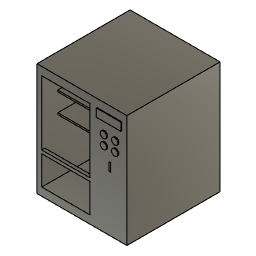
vendmachineprototype (Autodesk Fusion 360 design; units mm, degrees)
Autodesk Fusion 360 part; units mm, degrees
sketch "Sketch1" plane through (0, 0, 0) normal (0, 0, 1) x (1, 0, 0)
  line L0 (140, -145) -> (-140, -145)
  line L1 (-140, -145) -> (-140, 145)
  line L2 (-140, 145) -> (140, 145)
  line L3 (140, 145) -> (140, -145)
  line L4 (140, -145) -> (-140, 145) construction
  line L5 (-140, -145) -> (140, 145) construction
  dimension "d1" = 280
  dimension "d2" = 290
  constraint horizontal L0
  constraint perpendicular L0 L1
  constraint parallel L0 L2
  constraint parallel L1 L3
  constraint coincident L4 origin
  constraint coincident L5 origin
  measures "d1" distance of L1.end L2.end
  measures "d2" distance of L0.end L1.end
extrude "Extrude1" add sketch "Sketch1" along normal blind 350
sketch "Sketch2" plane through (0, -145, 0) normal (0, -1, 0) x (1, 0, 0)
  line L0 (-140, 0) -> (140, 0)
  line L1 (140, 0) -> (140, 350)
  line L2 (140, 350) -> (-140, 350)
  line L3 (-140, 350) -> (-140, 0)
  line L4 (25, 125) -> (-125, 125)
  line L5 (-125, 125) -> (-125, 325)
  line L6 (-125, 325) -> (25, 325)
  line L7 (25, 325) -> (25, 125)
  line L8 (25, 125) -> (-125, 325) construction
  line L9 (-125, 125) -> (25, 325) construction
  point P0 (-50, 225)
  constraint horizontal L4
  constraint perpendicular L4 L5
  constraint parallel L4 L6
  constraint parallel L5 L7
  constraint coincident L8 P0
  constraint coincident L9 P0
extrude "Extrude2" cut sketch "Sketch2" against normal blind 200 contours L4 L5 L6 L7
sketch "Sketch3" plane through (0, -145, 0) normal (0, -1, 0) x (1, 0, 0)
  line L0 (-125, 125) -> (-125, 325)
  line L1 (-125, 325) -> (25, 325)
  line L2 (25, 325) -> (25, 125)
  line L3 (25, 125) -> (-125, 125)
  line L4 (-140, 0) -> (140, 0)
  line L5 (140, 0) -> (140, 350)
  line L6 (140, 350) -> (-140, 350)
  line L7 (-140, 350) -> (-140, 0)
  line L8 (123.6698, 300.3073) -> (46.6698, 300.3073)
  line L9 (46.6698, 300.3073) -> (46.6698, 325.3073)
  line L10 (46.6698, 325.3073) -> (123.6698, 325.3073)
  line L11 (123.6698, 325.3073) -> (123.6698, 300.3073)
  line L12 (123.6698, 300.3073) -> (46.6698, 325.3073) construction
  line L13 (46.6698, 300.3073) -> (123.6698, 325.3073) construction
  circle A0 centre (70, 260) radius 9
  circle A1 centre (100, 260) radius 9
  circle A2 centre (70, 230) radius 9
  circle A3 centre (100, 230) radius 9
  line L14 (25, 22.9549) -> (-125, 22.9549)
  line L15 (-125, 22.9549) -> (-125, 112.9549)
  line L16 (-125, 112.9549) -> (25, 112.9549)
  line L17 (25, 112.9549) -> (25, 22.9549)
  line L18 (25, 22.9549) -> (-125, 112.9549) construction
  line L19 (-125, 22.9549) -> (25, 112.9549) construction
  line L20 (85, 185) -> (95, 185)
  line L21 (95, 185) -> (95, 160)
  line L22 (95, 160) -> (85, 160)
  line L23 (85, 160) -> (85, 185)
  point P0 (85.1698, 312.8073)
  point P1 (-50, 67.9549)
  dimension "d7" = 77
  dimension "d8" = 25
  dimension "d9" = 18
  dimension "d10" = 18
  dimension "d11" = 18
  dimension "d12" = 18
  dimension "d13" = 150
  dimension "d14" = 90
  constraint horizontal L8
  constraint perpendicular L8 L9
  constraint parallel L8 L10
  constraint parallel L9 L11
  constraint coincident L12 P0
  constraint coincident L13 P0
  constraint horizontal L14
  constraint perpendicular L14 L15
  constraint parallel L14 L16
  constraint parallel L15 L17
  constraint coincident L18 P1
  constraint coincident L19 P1
  constraint horizontal L20
  constraint vertical L21
  constraint horizontal L22
  constraint vertical L23
  measures "d7" distance of L9.end L10.end
  measures "d8" distance of L8.end L9.end
  measures "d9" diameter of A0
  measures "d10" diameter of A1
  measures "d11" diameter of A2
  measures "d12" diameter of A3
  measures "d13" distance of L15.end L16.end
  measures "d14" distance of L14.end L15.end
extrude "Extrude3" add sketch "Sketch3" along normal blind 2 contours L8 L9 L10 L11
sketch "Sketch4" plane through (0, 55, 0) normal (0, -1, 0) x (1, 0, 0)
  line L0 (25, 325) -> (-125, 325)
  line L1 (-125, 325) -> (-125, 125)
  line L2 (-125, 125) -> (25, 125)
  line L3 (25, 125) -> (25, 325)
  line L4 (-125, 200.3816) -> (25, 200.3816)
  line L5 (25, 200.3816) -> (25, 195.3816)
  line L6 (25, 195.3816) -> (-125, 195.3816)
  line L7 (-125, 195.3816) -> (-125, 200.3816)
  line L8 (-125, 261.7004) -> (25, 261.7004)
  line L9 (25, 261.7004) -> (25, 256.7004)
  line L10 (25, 256.7004) -> (-125, 256.7004)
  line L11 (-125, 256.7004) -> (-125, 261.7004)
  dimension "d17" = 5
  dimension "d18" = 150
  dimension "d19" = 5
  constraint horizontal L4
  constraint vertical L5
  constraint horizontal L6
  constraint vertical L7
  constraint coincident L1 L4.start
  constraint horizontal L8
  constraint vertical L9
  constraint horizontal L10
  constraint vertical L11
  constraint coincident L1 L8.start
  measures "d17" distance of L4.start L6.end
  measures "d18" distance of L8.start L8.end
  measures "d19" distance of L8.start L10.end
extrude "Extrude4" add sketch "Sketch4" along normal blind 150 contours L1 L3 L8 L9 L10 L11 | L1 L3 L4 L5 L6 L7
sketch "Sketch5" plane through (0, 0, 125) normal (0, 0, 1) x (-1, 0, 0)
  line L0 (125, 145) -> (-25, 145)
  line L1 (-25, 145) -> (-25, -55)
  line L2 (-25, -55) -> (125, -55)
  line L3 (125, -55) -> (125, 145)
  line L4 (-25, 135) -> (125, 135)
  line L5 (125, 135) -> (125, 5)
  line L6 (125, 5) -> (-25, 5)
  line L7 (-25, 5) -> (-25, 135)
  line L8 (-25, 135) -> (125, 5) construction
  line L9 (125, 135) -> (-25, 5) construction
  point P0 (50, 70)
  dimension "d22" = 130
  constraint horizontal L4
  constraint perpendicular L4 L5
  constraint parallel L4 L6
  constraint parallel L5 L7
  constraint coincident L8 P0
  constraint coincident L9 P0
  measures "d22" distance of L4.end L5.end
extrude "Extrude5" cut sketch "Sketch5" against normal blind 75 contours L1 L3 L4 L5 L6 L7
sketch "Sketch6" plane through (0, -145, 0) normal (0, -1, 0) x (1, 0, 0)
  line L0 (123.6698, 325.3073) -> (123.6698, 300.3073)
  line L1 (123.6698, 300.3073) -> (46.6698, 300.3073)
  line L2 (46.6698, 300.3073) -> (46.6698, 325.3073)
  line L3 (46.6698, 325.3073) -> (123.6698, 325.3073)
  line L4 (-125, 125) -> (-125, 325)
  line L5 (-125, 325) -> (25, 325)
  line L6 (25, 325) -> (25, 125)
  line L7 (25, 125) -> (-125, 125)
  line L8 (-140, 0) -> (140, 0)
  line L9 (140, 0) -> (140, 350)
  line L10 (140, 350) -> (-140, 350)
  line L11 (-140, 350) -> (-140, 0)
  line L12 (25, 25) -> (-125, 25)
  line L13 (-125, 25) -> (-125, 115)
  line L14 (-125, 115) -> (25, 115)
  line L15 (25, 115) -> (25, 25)
  line L16 (25, 25) -> (-125, 115) construction
  line L17 (-125, 25) -> (25, 115) construction
  point P0 (-50, 70)
  dimension "d25" = 150
  dimension "d26" = 90
  constraint horizontal L12
  constraint perpendicular L12 L13
  constraint parallel L12 L14
  constraint parallel L13 L15
  constraint coincident L16 P0
  constraint coincident L17 P0
  measures "d25" distance of L13.end L14.end
  measures "d26" distance of L12.end L13.end
extrude "Extrude6" cut sketch "Sketch6" against normal blind 150 contours L12 L13 L14 L15
sketch "Sketch7" plane through (0, -145, 0) normal (0, -1, 0) x (1, 0, 0)
  line L0 (-125, 25) -> (-125, 115)
  line L1 (-125, 115) -> (25, 115)
  line L2 (25, 115) -> (25, 25)
  line L3 (25, 25) -> (-125, 25)
  line L4 (123.6698, 325.3073) -> (123.6698, 300.3073)
  line L5 (123.6698, 300.3073) -> (46.6698, 300.3073)
  line L6 (46.6698, 300.3073) -> (46.6698, 325.3073)
  line L7 (46.6698, 325.3073) -> (123.6698, 325.3073)
  line L8 (-125, 125) -> (-125, 325)
  line L9 (-125, 325) -> (25, 325)
  line L10 (25, 325) -> (25, 125)
  line L11 (25, 125) -> (-125, 125)
  line L12 (-140, 0) -> (140, 0)
  line L13 (140, 0) -> (140, 350)
  line L14 (140, 350) -> (-140, 350)
  line L15 (-140, 350) -> (-140, 0)
  circle A0 centre (70, 265) radius 10
  circle A1 centre (105, 265) radius 10
  circle A2 centre (70, 235) radius 10
  circle A3 centre (105, 235) radius 10
  dimension "d29" = 20
  dimension "d30" = 20
  dimension "d31" = 20
  dimension "d32" = 20
  measures "d29" diameter of A0
  measures "d30" diameter of A1
  measures "d31" diameter of A2
  measures "d32" diameter of A3
extrude "Extrude7" add sketch "Sketch7" along normal blind 3 contours A0 | A1 | A2 | A3
sketch "Sketch8" plane through (0, -145, 0) normal (0, -1, 0) x (1, 0, 0)
  circle A0 centre (105, 235) radius 10
  circle A1 centre (70, 265) radius 10
  circle A2 centre (70, 235) radius 10
  circle A3 centre (105, 265) radius 10
  line L0 (-125, 25) -> (-125, 115)
  line L1 (-125, 115) -> (25, 115)
  line L2 (25, 115) -> (25, 25)
  line L3 (25, 25) -> (-125, 25)
  line L4 (123.6698, 325.3073) -> (123.6698, 300.3073)
  line L5 (123.6698, 300.3073) -> (46.6698, 300.3073)
  line L6 (46.6698, 300.3073) -> (46.6698, 325.3073)
  line L7 (46.6698, 325.3073) -> (123.6698, 325.3073)
  line L8 (-125, 125) -> (-125, 325)
  line L9 (-125, 325) -> (25, 325)
  line L10 (25, 325) -> (25, 125)
  line L11 (25, 125) -> (-125, 125)
  line L12 (-140, 0) -> (140, 0)
  line L13 (140, 0) -> (140, 350)
  line L14 (140, 350) -> (-140, 350)
  line L15 (-140, 350) -> (-140, 0)
  line L16 (89.5, 172) -> (84.5, 172)
  line L17 (84.5, 172) -> (84.5, 198)
  line L18 (84.5, 198) -> (89.5, 198)
  line L19 (89.5, 198) -> (89.5, 172)
  line L20 (89.5, 172) -> (84.5, 198) construction
  line L21 (84.5, 172) -> (89.5, 198) construction
  point P0 (87, 185)
  dimension "d35" = 5
  dimension "d36" = 26
  constraint horizontal L16
  constraint perpendicular L16 L17
  constraint parallel L16 L18
  constraint parallel L17 L19
  constraint coincident L20 P0
  constraint coincident L21 P0
  measures "d35" distance of L17.end L18.end
  measures "d36" distance of L16.end L17.end
extrude "Extrude8" cut sketch "Sketch8" against normal blind 100 contours L16 L17 L18 L19
